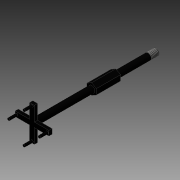
# Autodesk Inventor part: 杆件
Saved by Autodesk Inventor 2016 (Build 200138000, 138)
## iProperties
Created: 2019-04-01
Part Number: 杆件
Material: 常规
Document SubType Name: Modeling
Designer: oldboy
Density: 1 g/cm^3
Appearance: 默认
Author: oldboy
Autodesk Inventor part; units mm, degrees
ref_plane "YZ Plane" through (0, 0, 0) normal (1, 0, 0) x (0, 1, 0)
ref_plane "XZ Plane" through (0, 0, 0) normal (0, 1, 0) x (-1, 0, 0)
ref_plane "XY Plane" through (0, 0, 0) normal (0, 0, 1) x (1, 0, 0)
sketch "草图1" plane through (0, 0, 0) normal (0, 1, 0) x (-1, 0, 0)
  line L0 (2.95, -1.7032) -> (0, -3.4064)
  line L1 (0, -3.4064) -> (-2.95, -1.7032)
  line L2 (-2.95, -1.7032) -> (-2.95, 1.7032)
  line L3 (-2.95, 1.7032) -> (0, 3.4064)
  line L4 (0, 3.4064) -> (2.95, 1.7032)
  line L5 (2.95, 1.7032) -> (2.95, -1.7032)
  point P0 (0, 0)
  point P1 (0, 0)
  point P2 (2.95, 0)
  constraints: 12 end point, 1 midpoint, 13 other
extrude "拉伸1" add sketch "草图1" along normal blind 15
sketch "草图2" plane through (0, 15, 0) normal (0, 1, 0) x (1, 0, 0)
  circle A0 centre (0, 0) radius 1.95
  dimension "d3" = 3.9
  constraints: 1 centre point, 1 coincident
  measures "d3" diameter of A0
extrude "拉伸2" add sketch "草图2" along normal blind 25
thread "螺纹1" size "M4x0.7" class "6g" standard "ANSI Metric M Profile" length 5
sketch "草图6" plane through (0, 0, 0) normal (0, -1, 0) x (1, 0, 0)
  circle A0 centre (0, 0) radius 2
  dimension "d22" = 4
  constraints: 1 centre point, 1 coincident
  measures "d22" diameter of A0
extrude "拉伸6" add sketch "草图6" along normal blind 35
sketch "草图7" plane through (0, -35, 0) normal (0, -1, 0) x (1, 0, 0)
  line L0 (10.5, -1.5) -> (10.5, 1.5)
  line L1 (-10.5, 1.5) -> (-10.5, -1.5)
  line L2 (-10.5, -1.5) -> (10.5, 1.5) construction
  line L3 (10.5, -1.5) -> (-10.5, 1.5) construction
  line L4 (-1.5, 10.5) -> (1.5, 10.5)
  line L5 (1.5, -10.5) -> (-1.5, -10.5)
  line L6 (-1.5, 10.5) -> (1.5, -10.5) construction
  line L7 (1.5, 10.5) -> (-1.5, -10.5) construction
  line L8 (-1.5, 1.5) -> (-10.5, 1.5)
  line L9 (10.5, 1.5) -> (1.5, 1.5)
  line L10 (1.5, 10.5) -> (1.5, 1.5)
  line L11 (1.5, -1.5) -> (1.5, -10.5)
  line L12 (1.5, -1.5) -> (10.5, -1.5)
  line L13 (-10.5, -1.5) -> (-1.5, -1.5)
  line L14 (-1.5, -10.5) -> (-1.5, -1.5)
  line L15 (-1.5, 1.5) -> (-1.5, 10.5)
  point P0 (0, 0)
  dimension "d26" = 21
  constraints: 32 end point, 10 parallel, 5 perpendicular, 4 midpoint, 3 horizontal
  measures "d26" distance between parallel lines of L0 L1
extrude "拉伸7" add sketch "草图7" along normal blind 2
sketch "草图8" plane through (0, -37, 0) normal (0, -1, 0) x (1, 0, 0)
  circle A0 centre (0, 0) radius 9.5 construction
  circle A1 centre (0, 9.5) radius 0.75
  circle A2 centre (-9.5, 0) radius 0.75
  circle A3 centre (0, -9.5) radius 0.75
  circle A4 centre (9.5, 0) radius 0.75
  dimension "d29" = 19
  dimension "d30" = 1.5
  dimension "d31" = 1.5
  dimension "d32" = 1.5
  dimension "d33" = 1.5
  constraints: 5 centre point, 4 point on circle, 1 coincident
  measures "d29" diameter of A0
  measures "d30" diameter of A1
  measures "d31" diameter of A2
  measures "d32" diameter of A3
  measures "d33" diameter of A4
extrude "拉伸8" add sketch "草图8" along normal blind 5
